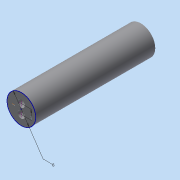
# Autodesk Inventor part: LED_support
Saved by Autodesk Inventor 2015 (Build 190159000, 159)
## iProperties
Created: 2015-02-02
Part Number: LED_support
Material: Generic
Document SubType Name: Modeling
Designer: Openlab
Density: 1 g/cm^3
Appearance: Default
Author: Openlab
Autodesk Inventor part; units mm, degrees
ref_plane "YZ Plane" through (0, 0, 0) normal (1, 0, 0) x (0, 1, 0)
ref_plane "XZ Plane" through (0, 0, 0) normal (0, 1, 0) x (-1, 0, 0)
ref_plane "XY Plane" through (0, 0, 0) normal (0, 0, 1) x (1, 0, 0)
sketch "Sketch1" plane through (0, 0, 0) normal (0, 1, 0) x (-1, 0, 0)
  circle A0 centre (0, 0) radius 3
  line L0 (1.3195, 0) -> (1.9456, 0) construction
  point P0 (0, 1)
  point P1 (0, -1)
  dimension "d0" = 6
  dimension "d1" = 2
  constraints: 2 end point, 1 centre point, 1 coincident, 1 horizontal, 1 symmetric about line, 1 vertical alignment
  measures "d0" diameter of A0
  measures "d1" distance of point (0, -1) point (0, 1)
extrude "Extrusion1" add sketch "Sketch1" along normal blind 25
hole "Hole1" at (0, 0, 1) at (0, 0, -1) direction (0, 1, 0) diameter 1.5 end through all
body "Solid1"
